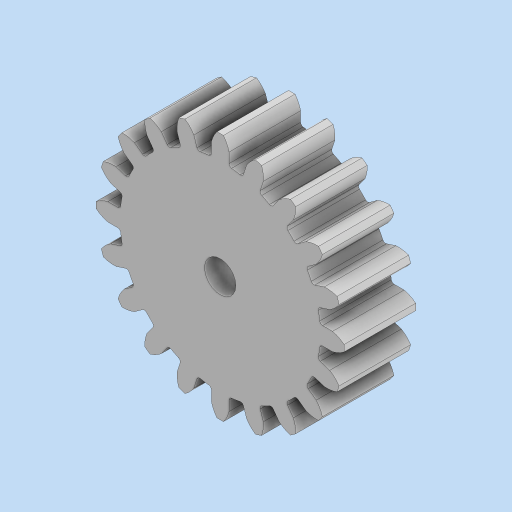
# Autodesk Inventor part: engrane
Saved by Autodesk Inventor 2024 (Build 280153000, 153)
## iProperties
Created: 2024-09-04
Part Number: engrane
Material: Generic
Document SubType Name: Modeling
Designer: MxMon
Density: 1 g/cm^3
Appearance: Default
Author: MxMon
Autodesk Inventor part; units mm, degrees
ref_plane "YZ Plane" through (0, 0, 0) normal (1, 0, 0) x (0, 1, 0)
ref_plane "XZ Plane" through (0, 0, 0) normal (0, 1, 0) x (-1, 0, 0)
ref_plane "XY Plane" through (0, 0, 0) normal (0, 0, 1) x (1, 0, 0)
sketch "Sketch1" plane through (0, 0, 0) normal (0, 0, 1) x (1, 0, 0)
  arc A0 (-1.5903, 13.9094) -> (1.5903, 13.9094) centre (0, 0) ccw
  arc A1 (1.2357, 15.7014) -> (-1.2357, 15.7014) centre (0, 0) ccw construction
  line L0 (0, 0) -> (-1.6646, 21.1512) construction
  line L1 (0, 0) -> (1.589, 20.1896) construction
  line L2 (0, 0) -> (0, 20.3411) construction
  arc A2 (0.45, 17.3192) -> (-0.45, 17.3192) centre (0, 0) ccw
  arc A3 (-0.45, 17.3192) -> (-1.2357, 15.7014) centre (2.6631, 14.8074) ccw
  arc A4 (1.2357, 15.7014) -> (0.45, 17.3192) centre (-2.6631, 14.8074) ccw
  line L3 (-1.2357, 15.7014) -> (-1.2357, 14.3068)
  line L4 (1.2357, 15.7014) -> (1.2357, 14.3068)
  arc A5 (-1.5903, 13.9094) -> (-1.2357, 14.3068) centre (-1.6357, 14.3068) ccw
  arc A6 (1.2357, 14.3068) -> (1.5903, 13.9094) centre (1.6357, 14.3068) ccw
  arc A7 (-4.9239, 16.6106) -> (-5.7799, 16.3324) centre (0, 0) ccw
  arc A8 (-5.8107, 12.7372) -> (-5.5963, 13.2247) centre (-5.9767, 13.1011) ccw
  line L5 (-6.0273, 14.5511) -> (-5.5963, 13.2247)
  arc A9 (-5.7799, 16.3324) -> (-6.0273, 14.5511) centre (-2.043, 14.9056) ccw
  arc A10 (-3.6768, 15.3148) -> (-4.9239, 16.6106) centre (-7.1085, 13.2598) ccw
  line L6 (-3.6768, 15.3148) -> (-3.2458, 13.9884)
  arc A11 (-3.2458, 13.9884) -> (-2.7858, 13.72) centre (-2.8654, 14.112) ccw
  arc A12 (-9.8159, 14.276) -> (-10.544, 13.747) centre (0, 0) ccw
  arc A13 (-9.4623, 10.3182) -> (-9.4091, 10.8481) centre (-9.7327, 10.613) ccw
  line L7 (-10.2288, 11.9764) -> (-9.4091, 10.8481)
  arc A14 (-10.544, 13.747) -> (-10.2288, 11.9764) centre (-6.5491, 13.5448) ccw
  arc A15 (-8.2294, 13.4291) -> (-9.8159, 14.276) centre (-10.8581, 10.4141) ccw
  line L8 (-8.2294, 13.4291) -> (-7.4096, 12.3008)
  arc A16 (-7.4096, 12.3008) -> (-6.8892, 12.1877) centre (-7.086, 12.5359) ccw
  arc A17 (-13.747, 10.544) -> (-14.276, 9.8159) centre (0, 0) ccw
  arc A18 (-12.1877, 6.8892) -> (-12.3008, 7.4096) centre (-12.5359, 7.086) ccw
  line L9 (-13.4291, 8.2294) -> (-12.3008, 7.4096)
  arc A19 (-14.276, 9.8159) -> (-13.4291, 8.2294) centre (-10.4141, 10.8581) ccw
  arc A20 (-11.9764, 10.2288) -> (-13.747, 10.544) centre (-13.5448, 6.5491) ccw
  line L10 (-11.9764, 10.2288) -> (-10.8481, 9.4091)
  arc A21 (-10.8481, 9.4091) -> (-10.3182, 9.4623) centre (-10.613, 9.7327) ccw
  arc A22 (-16.3324, 5.7799) -> (-16.6106, 4.9239) centre (0, 0) ccw
  arc A23 (-13.72, 2.7858) -> (-13.9884, 3.2458) centre (-14.112, 2.8654) ccw
  line L11 (-15.3148, 3.6768) -> (-13.9884, 3.2458)
  arc A24 (-16.6106, 4.9239) -> (-15.3148, 3.6768) centre (-13.2598, 7.1085) ccw
  arc A25 (-14.5511, 6.0273) -> (-16.3324, 5.7799) centre (-14.9056, 2.043) ccw
  line L12 (-14.5511, 6.0273) -> (-13.2247, 5.5963)
  arc A26 (-13.2247, 5.5963) -> (-12.7372, 5.8107) centre (-13.1011, 5.9767) ccw
  arc A27 (-17.3192, 0.45) -> (-17.3192, -0.45) centre (0, 0) ccw
  arc A28 (-13.9094, -1.5903) -> (-14.3068, -1.2357) centre (-14.3068, -1.6357) ccw
  line L13 (-15.7014, -1.2357) -> (-14.3068, -1.2357)
  arc A29 (-17.3192, -0.45) -> (-15.7014, -1.2357) centre (-14.8074, 2.6631) ccw
  arc A30 (-15.7014, 1.2357) -> (-17.3192, 0.45) centre (-14.8074, -2.6631) ccw
  line L14 (-15.7014, 1.2357) -> (-14.3068, 1.2357)
  arc A31 (-14.3068, 1.2357) -> (-13.9094, 1.5903) centre (-14.3068, 1.6357) ccw
  arc A32 (-16.6106, -4.9239) -> (-16.3324, -5.7799) centre (0, 0) ccw
  arc A33 (-12.7372, -5.8107) -> (-13.2247, -5.5963) centre (-13.1011, -5.9767) ccw
  line L15 (-14.5511, -6.0273) -> (-13.2247, -5.5963)
  arc A34 (-16.3324, -5.7799) -> (-14.5511, -6.0273) centre (-14.9056, -2.043) ccw
  arc A35 (-15.3148, -3.6768) -> (-16.6106, -4.9239) centre (-13.2598, -7.1085) ccw
  line L16 (-15.3148, -3.6768) -> (-13.9884, -3.2458)
  arc A36 (-13.9884, -3.2458) -> (-13.72, -2.7858) centre (-14.112, -2.8654) ccw
  arc A37 (-14.276, -9.8159) -> (-13.747, -10.544) centre (0, 0) ccw
  arc A38 (-10.3182, -9.4623) -> (-10.8481, -9.4091) centre (-10.613, -9.7327) ccw
  line L17 (-11.9764, -10.2288) -> (-10.8481, -9.4091)
  arc A39 (-13.747, -10.544) -> (-11.9764, -10.2288) centre (-13.5448, -6.5491) ccw
  arc A40 (-13.4291, -8.2294) -> (-14.276, -9.8159) centre (-10.4141, -10.8581) ccw
  line L18 (-13.4291, -8.2294) -> (-12.3008, -7.4096)
  arc A41 (-12.3008, -7.4096) -> (-12.1877, -6.8892) centre (-12.5359, -7.086) ccw
  arc A42 (-10.544, -13.747) -> (-9.8159, -14.276) centre (0, 0) ccw
  arc A43 (-6.8892, -12.1877) -> (-7.4096, -12.3008) centre (-7.086, -12.5359) ccw
  line L19 (-8.2294, -13.4291) -> (-7.4096, -12.3008)
  arc A44 (-9.8159, -14.276) -> (-8.2294, -13.4291) centre (-10.8581, -10.4141) ccw
  arc A45 (-10.2288, -11.9764) -> (-10.544, -13.747) centre (-6.5491, -13.5448) ccw
  line L20 (-10.2288, -11.9764) -> (-9.4091, -10.8481)
  arc A46 (-9.4091, -10.8481) -> (-9.4623, -10.3182) centre (-9.7327, -10.613) ccw
  arc A47 (-5.7799, -16.3324) -> (-4.9239, -16.6106) centre (0, 0) ccw
  arc A48 (-2.7858, -13.72) -> (-3.2458, -13.9884) centre (-2.8654, -14.112) ccw
  line L21 (-3.6768, -15.3148) -> (-3.2458, -13.9884)
  arc A49 (-4.9239, -16.6106) -> (-3.6768, -15.3148) centre (-7.1085, -13.2598) ccw
  arc A50 (-6.0273, -14.5511) -> (-5.7799, -16.3324) centre (-2.043, -14.9056) ccw
  line L22 (-6.0273, -14.5511) -> (-5.5963, -13.2247)
  arc A51 (-5.5963, -13.2247) -> (-5.8107, -12.7372) centre (-5.9767, -13.1011) ccw
  arc A52 (-0.45, -17.3192) -> (0.45, -17.3192) centre (0, 0) ccw
  arc A53 (1.5903, -13.9094) -> (1.2357, -14.3068) centre (1.6357, -14.3068) ccw
  line L23 (1.2357, -15.7014) -> (1.2357, -14.3068)
  arc A54 (0.45, -17.3192) -> (1.2357, -15.7014) centre (-2.6631, -14.8074) ccw
  arc A55 (-1.2357, -15.7014) -> (-0.45, -17.3192) centre (2.6631, -14.8074) ccw
  line L24 (-1.2357, -15.7014) -> (-1.2357, -14.3068)
  arc A56 (-1.2357, -14.3068) -> (-1.5903, -13.9094) centre (-1.6357, -14.3068) ccw
  arc A57 (4.9239, -16.6106) -> (5.7799, -16.3324) centre (0, 0) ccw
  arc A58 (5.8107, -12.7372) -> (5.5963, -13.2247) centre (5.9767, -13.1011) ccw
  line L25 (6.0273, -14.5511) -> (5.5963, -13.2247)
  arc A59 (5.7799, -16.3324) -> (6.0273, -14.5511) centre (2.043, -14.9056) ccw
  arc A60 (3.6768, -15.3148) -> (4.9239, -16.6106) centre (7.1085, -13.2598) ccw
  line L26 (3.6768, -15.3148) -> (3.2458, -13.9884)
  arc A61 (3.2458, -13.9884) -> (2.7858, -13.72) centre (2.8654, -14.112) ccw
  arc A62 (9.8159, -14.276) -> (10.544, -13.747) centre (0, 0) ccw
  arc A63 (9.4623, -10.3182) -> (9.4091, -10.8481) centre (9.7327, -10.613) ccw
  line L27 (10.2288, -11.9764) -> (9.4091, -10.8481)
  arc A64 (10.544, -13.747) -> (10.2288, -11.9764) centre (6.5491, -13.5448) ccw
  arc A65 (8.2294, -13.4291) -> (9.8159, -14.276) centre (10.8581, -10.4141) ccw
  line L28 (8.2294, -13.4291) -> (7.4096, -12.3008)
  arc A66 (7.4096, -12.3008) -> (6.8892, -12.1877) centre (7.086, -12.5359) ccw
  arc A67 (13.747, -10.544) -> (14.276, -9.8159) centre (0, 0) ccw
  arc A68 (12.1877, -6.8892) -> (12.3008, -7.4096) centre (12.5359, -7.086) ccw
  line L29 (13.4291, -8.2294) -> (12.3008, -7.4096)
  arc A69 (14.276, -9.8159) -> (13.4291, -8.2294) centre (10.4141, -10.8581) ccw
  arc A70 (11.9764, -10.2288) -> (13.747, -10.544) centre (13.5448, -6.5491) ccw
  line L30 (11.9764, -10.2288) -> (10.8481, -9.4091)
  arc A71 (10.8481, -9.4091) -> (10.3182, -9.4623) centre (10.613, -9.7327) ccw
  arc A72 (16.3324, -5.7799) -> (16.6106, -4.9239) centre (0, 0) ccw
  arc A73 (13.72, -2.7858) -> (13.9884, -3.2458) centre (14.112, -2.8654) ccw
  line L31 (15.3148, -3.6768) -> (13.9884, -3.2458)
  arc A74 (16.6106, -4.9239) -> (15.3148, -3.6768) centre (13.2598, -7.1085) ccw
  arc A75 (14.5511, -6.0273) -> (16.3324, -5.7799) centre (14.9056, -2.043) ccw
  line L32 (14.5511, -6.0273) -> (13.2247, -5.5963)
  arc A76 (13.2247, -5.5963) -> (12.7372, -5.8107) centre (13.1011, -5.9767) ccw
  arc A77 (17.3192, -0.45) -> (17.3192, 0.45) centre (0, 0) ccw
  arc A78 (13.9094, 1.5903) -> (14.3068, 1.2357) centre (14.3068, 1.6357) ccw
  line L33 (15.7014, 1.2357) -> (14.3068, 1.2357)
  arc A79 (17.3192, 0.45) -> (15.7014, 1.2357) centre (14.8074, -2.6631) ccw
  arc A80 (15.7014, -1.2357) -> (17.3192, -0.45) centre (14.8074, 2.6631) ccw
  line L34 (15.7014, -1.2357) -> (14.3068, -1.2357)
  arc A81 (14.3068, -1.2357) -> (13.9094, -1.5903) centre (14.3068, -1.6357) ccw
  arc A82 (16.6106, 4.9239) -> (16.3324, 5.7799) centre (0, 0) ccw
  arc A83 (12.7372, 5.8107) -> (13.2247, 5.5963) centre (13.1011, 5.9767) ccw
  line L35 (14.5511, 6.0273) -> (13.2247, 5.5963)
  arc A84 (16.3324, 5.7799) -> (14.5511, 6.0273) centre (14.9056, 2.043) ccw
  arc A85 (15.3148, 3.6768) -> (16.6106, 4.9239) centre (13.2598, 7.1085) ccw
  line L36 (15.3148, 3.6768) -> (13.9884, 3.2458)
  arc A86 (13.9884, 3.2458) -> (13.72, 2.7858) centre (14.112, 2.8654) ccw
  arc A87 (14.276, 9.8159) -> (13.747, 10.544) centre (0, 0) ccw
  arc A88 (10.3182, 9.4623) -> (10.8481, 9.4091) centre (10.613, 9.7327) ccw
  line L37 (11.9764, 10.2288) -> (10.8481, 9.4091)
  arc A89 (13.747, 10.544) -> (11.9764, 10.2288) centre (13.5448, 6.5491) ccw
  arc A90 (13.4291, 8.2294) -> (14.276, 9.8159) centre (10.4141, 10.8581) ccw
  line L38 (13.4291, 8.2294) -> (12.3008, 7.4096)
  arc A91 (12.3008, 7.4096) -> (12.1877, 6.8892) centre (12.5359, 7.086) ccw
  arc A92 (10.544, 13.747) -> (9.8159, 14.276) centre (0, 0) ccw
  arc A93 (6.8892, 12.1877) -> (7.4096, 12.3008) centre (7.086, 12.5359) ccw
  line L39 (8.2294, 13.4291) -> (7.4096, 12.3008)
  arc A94 (9.8159, 14.276) -> (8.2294, 13.4291) centre (10.8581, 10.4141) ccw
  arc A95 (10.2288, 11.9764) -> (10.544, 13.747) centre (6.5491, 13.5448) ccw
  line L40 (10.2288, 11.9764) -> (9.4091, 10.8481)
  arc A96 (9.4091, 10.8481) -> (9.4623, 10.3182) centre (9.7327, 10.613) ccw
  arc A97 (5.7799, 16.3324) -> (4.9239, 16.6106) centre (0, 0) ccw
  arc A98 (2.7858, 13.72) -> (3.2458, 13.9884) centre (2.8654, 14.112) ccw
  line L41 (3.6768, 15.3148) -> (3.2458, 13.9884)
  arc A99 (4.9239, 16.6106) -> (3.6768, 15.3148) centre (7.1085, 13.2598) ccw
  arc A100 (6.0273, 14.5511) -> (5.7799, 16.3324) centre (2.043, 14.9056) ccw
  line L42 (6.0273, 14.5511) -> (5.5963, 13.2247)
  arc A101 (5.5963, 13.2247) -> (5.8107, 12.7372) centre (5.9767, 13.1011) ccw
  point P0 (0, 17.325)
  point P1 (1.2357, 13.9454)
  point P2 (-1.2357, 13.9454)
  point P3 (-5.3537, 16.4771)
  point P4 (-10.1834, 14.0162)
  point P5 (-14.0162, 10.1834)
  point P6 (-16.4771, 5.3537)
  point P7 (-17.325, 0)
  point P8 (-16.4771, -5.3537)
  point P9 (-14.0162, -10.1834)
  point P10 (-10.1834, -14.0162)
  point P11 (-5.3537, -16.4771)
  point P12 (0, -17.325)
  point P13 (5.3537, -16.4771)
  point P14 (10.1834, -14.0162)
  point P15 (14.0162, -10.1834)
  point P16 (16.4771, -5.3537)
  point P17 (17.325, 0)
  point P18 (16.4771, 5.3537)
  point P19 (14.0162, 10.1834)
  point P20 (10.1834, 14.0162)
  point P21 (5.3537, 16.4771)
  point P22 (-2.7858, 13.72)
  point P23 (-5.8107, 12.7372)
  point P24 (-6.8892, 12.1877)
  point P25 (-12.1877, 6.8892)
  point P26 (-12.7372, 5.8107)
  point P27 (-12.7372, -5.8107)
  point P28 (-10.3182, -9.4623)
  point P29 (-9.4623, -10.3182)
  point P30 (-5.8107, -12.7372)
  point P31 (2.7858, -13.72)
  point P32 (5.8107, -12.7372)
  point P33 (9.4623, -10.3182)
  point P34 (10.3182, -9.4623)
  point P35 (12.7372, -5.8107)
  point P36 (13.72, 2.7858)
  point P37 (5.8107, 12.7372)
  dimension "d0" = 28
  dimension "d1" = 31.5
  dimension "d7" = 34.65
  dimension "d8" = 9
  dimension "d9" = 4.5
  dimension "d10" = 0.45
  dimension "d11" = 0.45
  dimension "d12" = 4
  dimension "d13" = 4
  dimension "d14" = 0.4
  dimension "d17" = 360
  constraints: 203 point on circle, 101 centre point, 86 end point, 4 coincident, 4 point on line, 3 vertical, 2 tangent, 1 equal radius, 429 other
  measures "d1" diameter of A1
  measures "d7" diameter of A2
  measures "d8" angle of L1 L0
  measures "d9" angle of L2 L0
  measures "d10" horizontal distance of point (0, 17.325) A2.end
  measures "d11" horizontal distance of A2.centre A2.start
  measures "d12" radius of A3
  measures "d13" radius of A4
  measures "d14" radius of A5
extrude "Extrusion1" add sketch "Sketch1" along normal blind 10
sketch "Sketch3" plane through (0, 0, 0) normal (0, 0, -1) x (-1, 0, 0)
  circle A0 centre (0, 0) radius 2.1875
  dimension "d31" = 4.375
  constraints: 1 centre point, 1 coincident
  measures "d31" diameter of A0
extrude "Extrusion3" cut sketch "Sketch3" against normal through all
sketch "Sketch5" plane through (0, 0, 0) normal (0, 0, -1) x (-1, 0, 0)
  line L0 (-6, 4) -> (6, 4)
  line L1 (6, 4) -> (6, -4)
  line L2 (6, -4) -> (-6, -4)
  line L3 (-6, -4) -> (-6, 4)
  line L4 (-6, 4) -> (6, -4) construction
  line L5 (6, 4) -> (-6, -4) construction
  point P0 (0, 0)
  dimension "d37" = 12
  dimension "d38" = 8
  constraints: 12 end point, 2 midpoint, 2 parallel, 1 horizontal, 1 perpendicular
  measures "d37" distance of L1.end L2.end
  measures "d38" distance of L0.end L1.end
extrude "Extrusion5" cut sketch "Sketch5" against normal blind 5
chamfer "Chamfer1" distance 2 angle 45 4 edges at (6, 4, 2.5) (-6, 4, 2.5) (6, -4, 2.5) (-6, -4, 2.5)
body "Solid1"
